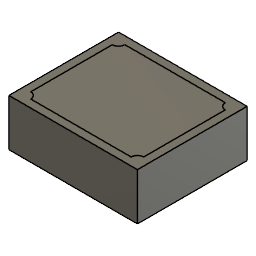
EnclosureBelow (Autodesk Fusion 360 design; units mm, degrees)
part number: 2026-09-07-18-19-06-847
Autodesk Fusion 360 part; units mm, degrees
sketch "Sketch3" plane through (0, 0, 0) normal (0, 1, 0) x (1, 0, 0)
  line L0 (41, -35) -> (-41, -35)
  line L1 (-41, -35) -> (-41, 35)
  line L2 (-41, 35) -> (41, 35)
  line L3 (41, 35) -> (41, -35)
  line L4 (41, -35) -> (-41, 35) construction
  line L5 (-41, -35) -> (41, 35) construction
  line L6 (36, -30) -> (-36, -30)
  line L7 (-36, -30) -> (-36, 30)
  line L8 (-36, 30) -> (36, 30)
  line L9 (36, 30) -> (36, -30)
  line L10 (36, -30) -> (-36, 30) construction
  line L11 (-36, -30) -> (36, 30) construction
  circle A0 centre (-36, 30) radius 4
  circle A1 centre (36, 30) radius 4
  circle A2 centre (-36, -30) radius 4
  circle A3 centre (36, -30) radius 4
  dimension "d16" = 82
  dimension "d17" = 70
  dimension "d18" = 60
  dimension "d19" = 72
  dimension "d20" = 8
  dimension "d21" = 8
  dimension "d22" = 8
  dimension "d23" = 8
  constraint horizontal L0
  constraint perpendicular L0 L1
  constraint parallel L0 L2
  constraint parallel L1 L3
  constraint coincident L4 origin
  constraint coincident L5 origin
  constraint horizontal L6
  constraint perpendicular L6 L7
  constraint parallel L6 L8
  constraint parallel L7 L9
  constraint coincident L10 origin
  constraint coincident L11 origin
  constraint coincident L7.end L8.start
  constraint coincident L8.end L9.start
  constraint coincident L6.end L7.start
  constraint coincident L6.start L9.end
  measures "d16" distance of L1.end L2.end
  measures "d17" distance of L0.start L2.end
  measures "d18" distance of L6.start L8.end
  measures "d19" distance of L7.end L8.end
  measures "d20" diameter of A0
  measures "d21" diameter of A1
  measures "d22" diameter of A2
  measures "d23" diameter of A3
extrude "Extrude2" add sketch "Sketch3" along normal blind 30 contours L0 L1 L2 L3 | L6 L7 A2 | L6 L7 A2 | L6 L9 A3 | L6 L9 A3 | L7 L8 A0 | L7 L8 A0 | L8 L9 A1 | L8 L9 A1 makes body 1
sketch "Sketch4" plane through (0, 30, 0) normal (0, 1, 0) x (-1, 0, 0)
  arc A0 (-32, -30) -> (-36, -26) centre (-36, -30) ccw
  line L0 (-36, -26) -> (-36, 26)
  arc A1 (-36, 26) -> (-32, 30) centre (-36, 30) ccw
  line L1 (-32, 30) -> (32, 30)
  arc A2 (32, 30) -> (36, 26) centre (36, 30) ccw
  line L2 (36, 26) -> (36, -26)
  arc A3 (36, -26) -> (32, -30) centre (36, -30) ccw
  line L3 (32, -30) -> (-32, -30)
  line L4 (-41, -35) -> (41, -35)
  line L5 (41, -35) -> (41, 35)
  line L6 (41, 35) -> (-41, 35)
  line L7 (-41, 35) -> (-41, -35)
  line L8 (37.9363, -31.7042) -> (-37.49, -31.7042)
  line L9 (-37.49, -31.7042) -> (-37.49, 33.0586)
  line L10 (-37.49, 33.0586) -> (37.9363, 33.0586)
  line L11 (37.9363, 33.0586) -> (37.9363, -31.7042)
  constraint horizontal L8
  constraint vertical L9
  constraint horizontal L10
  constraint vertical L11
extrude "Extrude3" add sketch "Sketch4" against normal blind 3 separate body contours A0 L0 A1 L1 A2 L2 A3 L3 makes body 2
sketch "Sketch5" plane through (0, 0, 0) normal (0, -1, 0) x (1, 0, 0)
  arc A0 (36, -26) -> (32, -30) centre (36, -30) ccw
  line L0 (32, -30) -> (-32, -30)
  arc A1 (-32, -30) -> (-36, -26) centre (-36, -30) ccw
  line L1 (-36, -26) -> (-36, 26)
  arc A2 (-36, 26) -> (-32, 30) centre (-36, 30) ccw
  line L2 (-32, 30) -> (32, 30)
  arc A3 (32, 30) -> (36, 26) centre (36, 30) ccw
  line L3 (36, 26) -> (36, -26)
  line L4 (-41, -35) -> (41, -35)
  line L5 (41, -35) -> (41, 35)
  line L6 (41, 35) -> (-41, 35)
  line L7 (-41, 35) -> (-41, -35)
  circle A4 centre (36, -30) radius 2.1
  circle A5 centre (-36, -30) radius 2.1
  circle A6 centre (36, 30) radius 2.1
  circle A7 centre (-36, 30) radius 2.1
  line L8 (36, -30) -> (-36, -30)
  line L9 (36, 30) -> (-36, 30)
  dimension "d28" = 4.2
  dimension "d29" = 4.2
  dimension "d30" = 4.2
  dimension "d31" = 4.2
  constraint concentric A0 A4
  constraint concentric A1 A5
  constraint concentric A3 A6
  constraint concentric A2 A7
  constraint coincident A0.centre A4.centre
  constraint coincident A1.centre A5.centre
  constraint coincident A3.centre A6.centre
  constraint coincident A2.centre A7.centre
  measures "d28" diameter of A4
  measures "d29" diameter of A5
  measures "d30" diameter of A7
  measures "d31" diameter of A6
extrude "Extrude4" cut sketch "Sketch5" against normal blind 5 contours A4 | A5 | A6 | A7 bodies 1
sketch "Sketch6" plane through (0, 27, 0) normal (0, -1, 0) x (1, 0, 0)
  line L0 (36, -26) -> (36, 26)
  arc A0 (32, 30) -> (36, 26) centre (36, 30) ccw
  line L1 (32, 30) -> (-32, 30)
  arc A1 (-36, 26) -> (-32, 30) centre (-36, 30) ccw
  line L2 (-36, 26) -> (-36, -26)
  arc A2 (-32, -30) -> (-36, -26) centre (-36, -30) ccw
  arc A3 (36, -26) -> (32, -30) centre (36, -30) ccw
  line L3 (-36, 32.5) -> (36, 32.5)
  line L4 (36, 32.5) -> (36, -32.5)
  line L5 (36, -32.5) -> (-36, -32.5)
  line L6 (-36, 32.5) -> (36, -32.5) construction
  line L7 (36, 32.5) -> (-36, -32.5) construction
  line L8 (-32, -30) -> (32, -30)
  dimension "d34" = 72
  dimension "d35" = 65
  constraint horizontal L3
  constraint perpendicular L3 L4
  constraint parallel L3 L5
  constraint coincident L6 origin
  constraint coincident L7 origin
  measures "d34" distance of L4.end L5.end
  measures "d35" distance of L3.start L5.end
sketch "Sketch7" plane through (0, 27, 0) normal (0, -1, 0) x (1, 0, 0)
  arc A0 (-32, -30) -> (-36, -26) centre (-36, -30) ccw
  line L0 (-32, -30) -> (32, -30)
  arc A1 (36, -26) -> (32, -30) centre (36, -30) ccw
  line L1 (36, -26) -> (36, 26)
  arc A2 (32, 30) -> (36, 26) centre (36, 30) ccw
  line L2 (32, 30) -> (-32, 30)
  arc A3 (-36, 26) -> (-32, 30) centre (-36, 30) ccw
  line L3 (-36, 26) -> (-36, -26)
  line L4 (34, -26.5) -> (-34, -26.5)
  line L5 (-34, -26.5) -> (-34, 26.5)
  line L6 (-34, 26.5) -> (34, 26.5)
  line L7 (34, 26.5) -> (34, -26.5)
  line L8 (34, -26.5) -> (-34, 26.5) construction
  line L9 (-34, -26.5) -> (34, 26.5) construction
  line L10 (34, 26.5) -> (31.46, 26.5)
  line L11 (34, 26.5) -> (31.5, 26.5)
  line L12 (31.5, 26.5) -> (31.5, -26.5)
  circle A4 centre (31.5, -19.5) radius 1.5
  circle A5 centre (31.5, 10.5) radius 1.5
  line L13 (-34, 26.5) -> (-34, 23.96)
  line L14 (-34, 23.96) -> (31.5, 23.96)
  circle A6 centre (-19, 23.96) radius 1.55
  dimension "d36" = 68
  dimension "d37" = 53
  dimension "d38" = 2.54
  dimension "d39" = 2.5
  dimension "d40" = 3
  dimension "d41" = 3
  dimension "d42" = 37
  dimension "d43" = 7
  dimension "d44" = 2.54
  dimension "d45" = 3.1
  dimension "d46" = 15
  constraint horizontal L4
  constraint perpendicular L4 L5
  constraint parallel L4 L6
  constraint parallel L5 L7
  constraint coincident L8 origin
  constraint coincident L9 origin
  constraint coincident L6 L10.end
  constraint coincident L10 L11.end
  constraint coincident L4 L12.end
  constraint perpendicular L4 L12
  constraint coincident L12 A4.centre
  constraint coincident L12 A5.centre
  constraint coincident L5 L13.end
  constraint coincident L12 L14.end
  constraint perpendicular L12 L14
  constraint coincident L14 A6.centre
  measures "d36" distance of L5.end L6.end
  measures "d37" distance of L4.start L6.end
  measures "d38" distance of L6.end L10.end
  measures "d39" distance of L4.start L12.end
  measures "d40" diameter of A5
  measures "d41" diameter of A4
  measures "d42" distance of L12.end A5.centre
  measures "d43" distance of L12.end A4.centre
  measures "d44" distance of L5.end L13.end
  measures "d45" diameter of A6
  measures "d46" distance of L13.end A6.centre
extrude "Extrude5" add sketch "Sketch7" along normal blind 6 contours L12 A4 | L12 A4 | L14 A6 | L14 A6 | L12 A5 | L12 A5 bodies 2
extrude "Extrude1" [suppressed]
sketch "Sketch2" plane through (0.0006, 0, 29) normal (0.00002, 0, 1) x (1, 0, -0.00002)
  line L0 (-39.9994, 0) -> (40.0006, 0)
  line L1 (40.0006, 0) -> (40.0006, 60)
  line L2 (40.0006, 60) -> (-39.9994, 60)
  line L3 (-39.9994, 60) -> (-39.9994, 0)
  line L4 (-35, 57.5) -> (35, 57.5)
  line L5 (35, 57.5) -> (35, 2.5)
  line L6 (35, 2.5) -> (-35, 2.5)
  line L7 (-35, 2.5) -> (-35, 57.5)
  line L8 (0, 0) -> (0.0006, 60)
  line L9 (0, 57.5) -> (0.0006, 60)
  dimension "d8" = 70
  dimension "d9" = 55
  dimension "d10" = 35
  dimension "d11" = 2.5
  dimension "d12" = 60
  constraint horizontal L4
  constraint vertical L5
  constraint horizontal L6
  constraint vertical L7
  constraint coincident L8.start origin
  constraint midpoint L2 L8.end
  constraint midpoint L4 L9.start
  measures "d8" distance of L4.start L4.end
  measures "d9" distance of L4.end L5.end
  measures "d10" distance of L6.end L8
  measures "d11" distance of L8.end L9.start
  measures "d12" distance of L0.end L1.end
